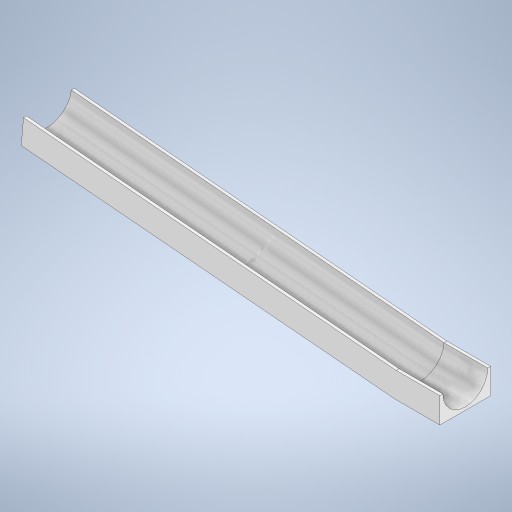
# Autodesk Inventor part: Conector superior para giro
Saved by Autodesk Inventor 2024 (Build 280153000, 153)
## iProperties
Created: 2023-05-11
Part Number: Conector superior para giro
Material: Plástico PET
Document SubType Name: Modeling
Designer: jpjoa
Density: 1.541 g/cm^3
Appearance: Branco
Author: jpjoa
Autodesk Inventor part; units mm, degrees
ref_plane "YZ Plane" through (0, 0, 0) normal (1, 0, 0) x (0, 1, 0)
ref_plane "XZ Plane" through (0, 0, 0) normal (0, 1, 0) x (-1, 0, 0)
sketch "Esboço1" plane through (0, 0, 0) normal (0, 0, 1) x (1, 0, 0)
  line L0 (150.4975, 10.2) -> (168.0522, 10.2)
  line L1 (150.4975, 10.2) -> (0.889, 23.2891)
  line L2 (168.0522, 1.2) -> (150.1046, 1.2)
  line L3 (150.1046, 1.2) -> (0.1046, 14.3233)
  line L4 (168.0522, 10.2) -> (168.0522, 0)
  line L5 (168.0522, 0) -> (150.0522, 0)
  line L6 (150.0522, 0) -> (0, 13.1279)
  line L7 (0, 13.1279) -> (0.889, 23.2891)
  point P0 (0, 0)
  dimension "d1" = 9
  dimension "d3" = 5
  dimension "d5" = 150
  dimension "d6" = 1.2
  dimension "d7" = 18
  constraints: 16 end point, 2 point on line, 2 vertical alignment, 1 horizontal, 1 horizontal alignment, 1 perpendicular, 2 other
  measures "d1" distance between parallel lines of L0 L2
  measures "d3" angle of L3 L2
  measures "d5" horizontal distance of L2.end L3.end
  measures "d6" distance between parallel lines of L3 L6
  measures "d7" distance of L4.end L5.end
extrude "Extrusão1" add sketch "Esboço1" along normal mid plane 20.4
ref_plane "Plano de trabalho2" through (0, 0, 0) normal (0, 0, 1) x (1, 0, 0)
sketch "Esboço3" plane through (0, 0, 0) normal (0, 0, 1) x (1, 0, 0)
  line L0 (0.889, 23.2891) -> (150.4975, 10.2)
  line L1 (150.4975, 10.2) -> (168.0522, 10.2)
  line L2 (0.1046, 14.3233) -> (150.1046, 1.2)
  line L3 (150.1046, 1.2) -> (168.0522, 1.2)
  line L4 (168.0522, 10.2) -> (168.0522, 1.2)
  line L5 (0.889, 23.2891) -> (0.1046, 14.3233)
  line L6 (0, 13.1279) -> (0.889, 23.2891) projected
  point P0 (0, 0)
  point P1 (150.4975, 10.2)
  dimension "d10" = 9
  constraints: 12 end point, 5 coincident, 1 collinear, 1 horizontal, 1 perpendicular, 1 other
  measures "d10" distance between parallel lines of L0 L2
extrude "Extrusão2" cut sketch "Esboço3" along normal mid plane 18
fillet "Arredondamento1" radius 9 4 edges at (75.1046, 7.7616, -9) (159.0784, 1.2, -9) (75.1046, 7.7616, 9) (159.0784, 1.2, 9)
equation "\"d1\" = 0.5 * Diâmetro_esfera"
equation "\"d6\" = Margem"
equation "\"d7\" = Diâmetro_esfera"
equation "\"d8\" = Diâmetro_esfera + 2 * Margem"
equation "\"d10\" = 0.5 * Diâmetro_esfera"
equation "\"d11\" = Diâmetro_esfera"
equation "\"d13\" = 0.5 * Diâmetro_esfera"
equation "\"Diâmetro_esfera\" = 18"
equation "\"Filamento\" = 0.4"
equation "\"Margem\" = 3 * Filamento"
